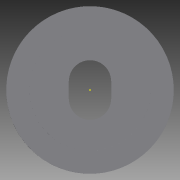
# Autodesk Inventor part: bracket
Saved by Autodesk Inventor 2015 SP2 (Build 190223200, 223)
## iProperties
Created: 2016-02-24
Part Number: bracket
Material: Generic
Document SubType Name: Modeling
Designer: Brandon
Density: 1 g/cm^3
Appearance: Default
Author: Brandon
Autodesk Inventor part; units mm, degrees
ref_plane "YZ Plane" through (0, 0, 0) normal (1, 0, 0) x (0, 1, 0)
ref_plane "XZ Plane" through (0, 0, 0) normal (0, 1, 0) x (-1, 0, 0)
ref_plane "XY Plane" through (0, 0, 0) normal (0, 0, 1) x (1, 0, 0)
sketch "Sketch1" plane through (0, 0, 0) normal (0, 0, 1) x (1, 0, 0)
  circle A0 centre (0, 0) radius 15.75
  circle A1 centre (0, 0) radius 21.75
  dimension "d1" = 31.5
  dimension "d2" = 43.5
  constraints: 2 centre point, 1 coincident
  measures "d1" diameter of A0
  measures "d2" diameter of A1
extrude "Extrusion1" add sketch "Sketch1" along normal blind 6.35 contours A0 | A1
sketch "Sketch2" plane through (0, 0, 6.35) normal (0, 0, 1) x (1, 0, 0)
  circle A0 centre (0, 0) radius 21.75
  circle A1 centre (0, 0) radius 15.75
  dimension "d5" = 31.5
  constraints: 2 centre point, 2 coincident
  measures "d5" diameter of A1
extrude "Extrusion2" add sketch "Sketch2" along normal blind 6.35
sketch "Sketch3" plane through (0, 0, 6.35) normal (0, 0, 1) x (1, 0, 0)
  line L0 (0, -4.75) -> (0, -8.25)
  line L1 (0, -8.25) -> (0, -4.75)
  line L2 (0, 4.75) -> (0, 8.25)
  line L3 (0, 0) -> (0, -1.75)
  line L4 (0, 0) -> (0, 1.75)
  line L5 (0, 0) -> (0, 2.25)
  line L6 (0, 0) -> (0, -2.25)
  line L7 (4.7631, 0) -> (0, 0)
  arc A0 (-5.5, -2.25) -> (5.5, -2.25) centre (0, -2.25) ccw
  arc A1 (5.5, 2.25) -> (-5.5, 2.25) centre (0, 2.25) ccw
  line L8 (-5.5, 2.25) -> (-5.5, -2.25)
  line L9 (5.5, 2.25) -> (5.5, -2.25)
  point P0 (-5.5102, 0)
  dimension "d11" = 8.25
  dimension "d12" = 8.25
  dimension "d32" = 2.25
  dimension "d33" = 2.25
  constraints: 20 end point, 4 point on circle, 4 vertical, 3 point on line, 2 centre point, 2 coincident, 2 tangent, 1 collinear
  measures "d11" distance of L3.start L0.end
  measures "d12" distance of L3.start L2.end
  measures "d32" distance of L3.start L5.end
  measures "d33" distance of L3.start L6.end
extrude "Extrusion3" cut sketch "Sketch3" along normal through all both and the other way through all
sketch "Sketch4" plane through (0, 0, 12.7) normal (0, 0, 1) x (1, 0, 0)
  point P0 (0, 0)
sketch "Sketch5" plane through (0, 0, 12.7) normal (0, 0, 1) x (1, 0, 0)
  circle A0 centre (0, 0) radius 15.75 projected
  line L0 (0, 15.75) -> (0, 21.75)
  circle A1 centre (0, 0) radius 21.75 projected
  line L1 (-14.7967, 5.3964) -> (-20.2679, 7.8914)
  arc A2 (0, 15.75) -> (-14.7967, 5.3964) centre (0, 0) ccw
  arc A3 (0, 21.75) -> (-20.2679, 7.8914) centre (0, 0) ccw
  constraints: 8 point on circle, 4 end point, 2 centre point, 2 concentric, 1 vertical
extrude "Extrusion4" cut sketch "Sketch5" against normal blind 6.35 contours A0 L1 A1 L0 picked at (-1.7226, 19.5424)
sketch "Sketch6" plane through (0, 0, 12.7) normal (0, 0, 1) x (1, 0, 0)
  point P0 (0, 0)
sketch "Sketch7" plane through (0, 0, 12.7) normal (0, 0, 1) x (1, 0, 0)
  circle A0 centre (0, 0) radius 21.75
  circle A1 centre (0, 0) radius 15.75
  constraints: 2 centre point, 2 coincident
extrude "Extrusion5" add sketch "Sketch7" against normal blind 6.35
sketch "Sketch8" plane through (0, 0, 12.7) normal (0, 0, 1) x (1, 0, 0)
  point P0 (0, 0)
sketch "Sketch9" plane through (0, 0, 12.7) normal (0, 0, 1) x (1, 0, 0)
  circle A0 centre (0, 0) radius 15.75
  circle A1 centre (0, 0) radius 21.75
  circle A2 centre (0, 0) radius 21.75 projected
  circle A3 centre (0, 0) radius 15.75 projected
  line L0 (15.7497, -0.1038) -> (21.6454, 2.1307)
  arc A4 (15.7497, -0.1038) -> (0, 15.75) centre (0, 0) ccw
  arc A5 (21.6454, 2.1307) -> (2.0753, 21.6508) centre (0, 0) ccw
  line L1 (0, 15.75) -> (0.0466, 21.7499)
  circle A6 centre (0, 0) radius 21.75 projected
  arc A7 (21.6454, 2.1307) -> (0.0466, 21.7499) centre (0, 0) ccw
  constraints: 13 point on circle, 5 centre point, 4 end point, 2 coincident, 1 concentric, 5 other
extrude "Extrusion6" cut sketch "Sketch9" against normal blind 6.35 contours A0 L1 A1 L0 picked at (4.1755, 19.2056)
sketch "Sketch10" plane through (0, 0, 12.7) normal (0, 0, 1) x (1, 0, 0)
  circle A0 centre (0, 0) radius 15.75
  circle A1 centre (0, 0) radius 21.75
  point P0 (15.7497, -0.1038)
  constraints: 2 coincident, 1 centre point, 3 other
extrude "Extrusion7" add sketch "Sketch10" along normal blind 6.35
sketch "Sketch11" plane through (0, 0, 19.05) normal (0, 0, 1) x (1, 0, 0)
  circle A0 centre (0, 0) radius 21.75 projected
  circle A1 centre (0, 0) radius 15.75
  circle A2 centre (0, 0) radius 21.75
  arc A3 (0, 15.75) -> (15.7497, -0.1038) centre (0, 0) ccw projected
  line L0 (12.1903, -9.9729) -> (16.8342, -13.7721)
  line L1 (-12.1903, 9.9729) -> (-16.8342, 13.7721)
  arc A4 (12.1903, -9.9729) -> (-12.1903, 9.9729) centre (0, 0) ccw
  arc A5 (16.8342, -13.7721) -> (-16.8342, 13.7721) centre (0, 0) ccw
  line L2 (-12.1903, 9.9729) -> (-16.8342, 13.7721)
  line L3 (12.1903, -9.9729) -> (16.8342, -13.7721)
  arc A6 (12.1903, -9.9729) -> (-12.1903, 9.9729) centre (0, 0) ccw
  point P0 (6.5, 1.75)
  point P1 (-6.5, 1.75)
  constraints: 8 end point, 8 point on circle, 3 centre point, 2 coincident, 1 collinear, 1 concentric, 8 other
extrude "Extrusion8" cut sketch "Sketch11" against normal blind 6.35 contours A0 L0 A1 L1 picked at (19.4008, 2.9309)
body "Solid1"
